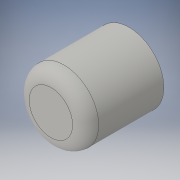
# Autodesk Inventor part: MetalFrame
Saved by Autodesk Inventor 2016 (Build 200138000, 138)
## iProperties
Created: 2017-12-19
Part Number: MetalFrame
Material: Generic
Document SubType Name: Modeling
Designer: Student
Density: 1 g/cm^3
Appearance: Default
Author: Student
Autodesk Inventor part; units mm, degrees
ref_plane "YZ Plane" through (0, 0, 0) normal (1, 0, 0) x (0, 1, 0)
ref_plane "XZ Plane" through (0, 0, 0) normal (0, 1, 0) x (-1, 0, 0)
ref_plane "XY Plane" through (0, 0, 0) normal (0, 0, 1) x (1, 0, 0)
sketch "Sketch1" plane through (0, 0, 0) normal (0, 0, 1) x (1, 0, 0)
  circle A0 centre (0, 0) radius 20.32
  dimension "d0" = 40.64
  constraints: 1 centre point, 1 coincident
  measures "d0" diameter of A0
extrude "Extrusion1" add sketch "Sketch1" along normal blind 45.72
sketch "Sketch2" plane through (0, 0, 0) normal (0, 0, -1) x (-1, 0, 0)
  circle A0 centre (0, 0) radius 19.05
  circle A1 centre (0, 0) radius 20.32 projected
  dimension "d3" = 38.1
  constraints: 1 centre point, 1 concentric
  measures "d3" diameter of A0
extrude "Extrusion2" cut sketch "Sketch2" against normal blind 40.64 contours A0
sketch "Sketch3" plane through (0, 0, 40.64) normal (0, 0, -1) x (-1, 0, 0)
  arc A0 (16.51, 2.54) -> (16.51, -2.54) centre (16.51, 0) ccw
  circle A1 centre (0, 0) radius 19.05 projected
  line L0 (16.51, 2.54) -> (18.8799, 2.54)
  line L1 (16.51, -2.54) -> (18.8799, -2.54)
  arc A2 (18.8799, -2.54) -> (18.8799, 2.54) centre (0, 0) ccw
  line L2 (2.6862, 16.4868) -> (3.4185, 18.7408)
  arc A3 (8.2499, 17.171) -> (3.4185, 18.7408) centre (0, 0) ccw
  line L3 (7.5176, 14.917) -> (8.2499, 17.171)
  arc A4 (2.6862, 16.4868) -> (7.5176, 14.917) centre (5.1019, 15.7019) ccw
  line L4 (-14.8498, 7.6494) -> (-16.7671, 9.0424)
  arc A5 (-13.7812, 13.1522) -> (-16.7671, 9.0424) centre (0, 0) ccw
  line L5 (-11.8639, 11.7592) -> (-13.7812, 13.1522)
  arc A6 (-14.8498, 7.6494) -> (-11.8639, 11.7592) centre (-13.3569, 9.7043) ccw
  line L6 (-11.8639, -11.7592) -> (-13.7812, -13.1522)
  arc A7 (-16.7671, -9.0424) -> (-13.7812, -13.1522) centre (0, 0) ccw
  line L7 (-14.8498, -7.6494) -> (-16.7671, -9.0424)
  arc A8 (-11.8639, -11.7592) -> (-14.8498, -7.6494) centre (-13.3569, -9.7043) ccw
  line L8 (7.5176, -14.917) -> (8.2499, -17.171)
  arc A9 (3.4185, -18.7408) -> (8.2499, -17.171) centre (0, 0) ccw
  line L9 (2.6862, -16.4868) -> (3.4185, -18.7408)
  arc A10 (7.5176, -14.917) -> (2.6862, -16.4868) centre (5.1019, -15.7019) ccw
  dimension "d6" = 5.08
  dimension "d9" = 360
  constraints: 22 point on circle, 20 end point, 10 centre point, 3 tangent, 2 horizontal, 1 concentric, 1 horizontal alignment, 51 other
  measures "d6" diameter of A0
extrude "Extrusion3" add sketch "Sketch3" along normal up to surface (40.64 mm away) contours L0 A1 L1 A0 | L3 A4 L2 A1 | A1 L9 A10 L8 | L5 A6 L4 A1 | A1 L7 A8 L6
sketch "Sketch4" plane through (0, 0, 0) normal (0, 0, -1) x (-1, 0, 0)
  arc A0 (16.51, 2.54) -> (16.51, -2.54) centre (16.51, 0) ccw projected
  circle A1 centre (16.51, 0) radius 1.524
  circle A2 centre (5.1019, 15.7019) radius 1.524
  circle A3 centre (-13.3569, 9.7043) radius 1.524
  circle A4 centre (-13.3569, -9.7043) radius 1.524
  circle A5 centre (5.1019, -15.7019) radius 1.524
  point P0 (0, 0)
  dimension "d13" = 3.048
  dimension "d16" = 360
  constraints: 5 centre point, 1 coincident, 11 other
  measures "d13" diameter of A1
extrude "Extrusion4" cut sketch "Sketch4" against normal blind 33.02
fillet "Fillet1" radius 7.62 1 edges at (-20.32, 0, 45.72)
fillet "Fillet2" radius 3.175 1 edges at (-18.8799, -2.54, 20.32)
body "Solid1"
